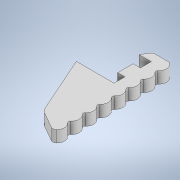
# Autodesk Inventor part: snow_feets
Saved by Autodesk Inventor 2020 (Build 240168000, 168)
## iProperties
Created: 2019-11-27
Part Number: snow_feets
Material: Generic
Document SubType Name: Modeling
Designer: erwin
Density: 1 g/cm^3
Appearance: Default
Author: erwin
Autodesk Inventor part; units mm, degrees
ref_plane "YZ Plane" through (0, 0, 0) normal (1, 0, 0) x (0, 1, 0)
ref_plane "XZ Plane" through (0, 0, 0) normal (0, 1, 0) x (-1, 0, 0)
ref_plane "XY Plane" through (0, 0, 0) normal (0, 0, 1) x (1, 0, 0)
sketch "Sketch1" plane through (0, 0, 0) normal (0, 1, 0) x (-1, 0, 0)
  line L0 (0, 0) -> (0, 120)
  line L1 (0, 120) -> (21, 108)
  line L2 (21, 108) -> (47.5, 48)
  line L3 (47.5, 48) -> (9, 48)
  line L4 (9, 48) -> (9, 36)
  line L5 (9, 36) -> (14, 36)
  line L6 (14, 36) -> (14, 20)
  line L7 (14, 20) -> (9, 20)
  line L8 (9, 20) -> (9, 8)
  line L9 (9, 8) -> (21, 8)
  line L10 (0, 0) -> (16.3812, 0)
  line L11 (16.3812, 0) -> (21, 8)
  dimension "d0" = 12
  dimension "d1" = 12
  dimension "d2" = 40
  dimension "d3" = 5
  dimension "d4" = 9
  dimension "d5" = 38.5
  dimension "d6" = 8
  dimension "d7" = 120
  dimension "d8" = 21
  dimension "d9" = 60
  dimension "d10" = 12
  dimension "d13" = 12
  constraints: 24 end point, 5 perpendicular, 2 point on line, 1 horizontal, 1 vertical
  measures "d0" distance of L7.end L8.end
  measures "d1" distance of L3.end L4.end
  measures "d2" distance between parallel lines of L9 L3
  measures "d3" distance between parallel lines of L4 L6
  measures "d4" distance between parallel lines of L8 L0
  measures "d5" distance of L2.end L3.end
  measures "d6" distance from line of L0.start L9
  measures "d7" distance of L0.start L0.end
  measures "d8" distance from line of L0 L1.end
  measures "d9" angle of L10 L11
  measures "d10" distance from line of L8 L9.end
  measures "d13" vertical distance of L0.end L1.end
extrude "Extrusion1" add sketch "Sketch1" along normal blind 12
sketch "Sketch2" plane through (0, 0, 0) normal (0, -1, 0) x (1, 0, 0)
  line L0 (0, 120) -> (0, 0) projected
  arc A0 (0, 0) -> (0, 15) centre (-2.7839, 7.5) ccw
  arc A1 (0, 15) -> (0, 30) centre (-2.7839, 22.5) ccw
  arc A2 (0, 30) -> (0, 45) centre (-2.7839, 37.5) ccw
  arc A3 (0, 45) -> (0, 60) centre (-2.7839, 52.5) ccw
  arc A4 (0, 60) -> (0, 75) centre (-2.7839, 67.5) ccw
  arc A5 (0, 75) -> (0, 90) centre (-2.7839, 82.5) ccw
  arc A6 (0, 90) -> (0, 105) centre (-2.7839, 97.5) ccw
  arc A7 (0, 105) -> (0, 120) centre (-2.7839, 112.5) ccw
  point P0 (0, 105)
  point P1 (0, 105)
  point P2 (0, 105)
  point P3 (0, 90)
  point P4 (0, 90)
  point P5 (0, 90)
  point P6 (0, 75)
  point P7 (0, 75)
  point P8 (0, 75)
  point P9 (0, 60)
  point P10 (0, 60)
  point P11 (0, 60)
  point P12 (0, 45)
  point P13 (0, 45)
  point P14 (0, 45)
  point P15 (0, 30)
  point P16 (0, 30)
  point P17 (0, 30)
  point P18 (0, 15)
  point P19 (0, 15)
  dimension "d14" = 8
  dimension "d15" = 15
  dimension "d18" = 15
  constraints: 16 point on circle, 8 centre point, 1 point on line, 1 vertical, 28 other
  measures "d14" radius of A0
  measures "d15" distance of L0.end A0.end
  measures "d18" distance of A0.centre A1.centre
extrude "Extrusion2" add sketch "Sketch2" against normal blind 12
fillet "Fillet1" radius 2 7 edges at (0, 6, 15) (0, 6, 30) (0, 6, 45) (0, 6, 60) (0, 6, 75) (0, 6, 90) (0, 6, 105)
fillet "Fillet1" radius 4 3 edges at (0, 6, 120) (0, 6, 0) (-16.3812, 6, 0)
fillet "Fillet1" radius 10 1 edges at (-21, 6, 108)
move faces "Move1" translate (0, 0, -0.8) faces at (-21.8333, 4, 48)
move faces "Move2" translate (0, 0, 0.8) faces at (-17, 4, 8)
move faces "Move3" translate (-2.5, 0, 0) faces at (-14, 4, 25.3333)
equation "\"d8\" = d4 + d10"
equation "\"d15\" = 0.125 * d7"
equation "\"d18\" = d15"
body "Solid1"
